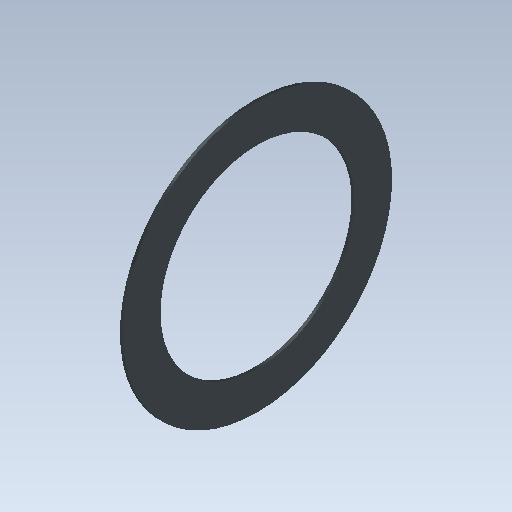
# Autodesk Inventor part: 6900ZZst
Saved by Autodesk Inventor 2021 (Build 250183000, 183)
## iProperties
Category: PARTsolutions
Company: NTN
Created: 2019-07-31
Part Number: 6900ZZst
Material: 鉄、鋳鉄
Catalog Web Link: www.cadenas.de
Description: Open type st-Deep Groove Ball Bearings
Vendor: NTN
Document SubType Name: Modeling
Designer: psadmin
Manufacturer: NTN
Mass: 0.204051 g
Surface Area: 3.00982 cm^2
Volume: 0.0285385 cm^3
Density: 7.15 g/cm^3
Appearance: 鉄 灰色
PSOL_IDENT_0: {$CADENAS_DATA\23d-libs\ntn\ball_roller_bearings\deep_groove_bb\deep_groove_bb\6_types\dgbb_st.prj},
PSOL_IDENT_1: 164 {VTYP=3D},{NB=6900ZZst},{LINA=6900ZZst},{NN=Open type st},{DATE=29.01.2019 23:03:44},{GEOMDATE=1
PSOL_IDENT_2: 4.01.2008 00:00:00},{VERSION=},{LINEID=2800},{WBVAR=},{WBNUMERIC=}  {NB=6900ZZst},{LINA=6900ZZst},{K
PSOL_IDENT_3: T=DUMMY},{IDNR=},{SD=10},{D=22},{B=6},{R=0.3},{ORDER1=6900},{ORDER=6900ZZ},{CR=2.70},{COR=1.27},{CRF=
PSOL_IDENT_4: 275},{CORF=129},{LSG=30000},{LSO=36000},{MASS=0.01},{RNS=0.3},{LLH=0},{LLU=21000},{ST=ZZ},{NCST=LLB}
PSOL_IDENT_5: ,{LTST=0},{CST=LLU},{SRG=N},{SR=NR},{D1=20.80},{A=1.05},{BA=0.80},{R0=0.20},{D2=24.8},{F=0.70},{DA1=
PSOL_IDENT_6: 12},{DA2=13},{DA=20},{DX=25.5},{CY=1.5},{CZ=0.7},{RAS=0.3},{RNAS=0.3},{VERS=2},{X=6}
NN: Open type st
NT: Deep Groove Ball Bearings
NB: 6900ZZst
NBSYN: $ORDER.st
LINA: 6900ZZst
SD: 10
D: 22
B: 6
R: 0.3
ORDER1: 6900
CR: 2.70
COR: 1.27
CRF: 275
CORF: 129
LSG: 30000
LSO: 36000
MASS: 0.01
RNS: 0.3
LLH: 0
LLU: 21000
ST: ZZ
NCST: LLB
LTST: 0
CST: LLU
SRG: N
SR: NR
D1: 20.8
A: 1.05
BA: 0.8
R0: 0.2
D2: 24.8
F: 0.7
DA1: 12
DA2: 13
DA: 20
DX: 25.5
CY: 1.5
CZ: 0.7
RAS: 0.3
RNAS: 0.3
VERS: 2
SUPPLIER: NTN
ARTICLENO: 6900ZZst
BOMINFO: 6900ZZst
CREATOR: CADENAS GmbH
Title: 6900ZZst
Author: Cadenas PARTsolutions
Comments: Deep Groove Ball Bearings
Autodesk Inventor part; units mm, degrees
sketch "Sketch_1" plane through (0, 0, 0) normal (0, 0, 1) x (1, 0, 0)
  line L0 (0.276, 0) -> (0.072, 0)
  line L1 (0.072, 9.6133) -> (0.072, 6.92)
  line L2 (0.072, 6.92) -> (0.276, 6.92)
  line L3 (0.276, 6.92) -> (0.276, 9.6133)
  line L4 (0.276, 9.6133) -> (0.072, 9.6133)
  constraints: 10 end point
revolve "Revolution1" add sketch "Sketch_1" angle 360 about axis through (0.276, 0, 0) along (1, 0, 0)
ref_plane "dgbb_st_XY" through (0, 0, 0) normal (1, 0, 0) x (0, 0, -1)
ref_plane "dgbb_st_YZ" through (0, 0, 0) normal (0, 0, -1) x (0, 1, 0)
ref_plane "dgbb_st_ZX" through (0, 0, 0) normal (0, 1, 0) x (1, 0, 0)
body "Solid1"
